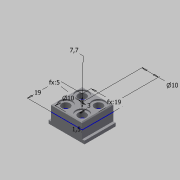
# Autodesk Inventor part: Bumper_button
Saved by Autodesk Inventor 2019.3 (Build 233278000, 278)
## iProperties
Created: 2019-02-26
Part Number: Bumper_button
Material: Generic
Document SubType Name: Modeling
Designer: Varga Daniel
Density: 1 g/cm^3
Appearance: Default
Author: Varga Daniel
Autodesk Inventor part; units mm, degrees
ref_plane "YZ Plane" through (0, 0, 0) normal (1, 0, 0) x (0, 1, 0)
ref_plane "XZ Plane" through (0, 0, 0) normal (0, 1, 0) x (-1, 0, 0)
ref_plane "XY Plane" through (0, 0, 0) normal (0, 0, 1) x (1, 0, 0)
derived "Base_part.ipt"
sketch "Beam_sketch" plane through (0, 0, 0) normal (0, 1, 0) x (-1, 0, 0)
  line L0 (5, 0) -> (25, 0)
  line L1 (30, 5) -> (30, 25)
  line L2 (25, 30) -> (5, 30)
  line L3 (0, 25) -> (0, 5)
  line L4 (5, 29) -> (25, 29)
  line L5 (29, 25) -> (29, 5)
  line L6 (25, 1) -> (5, 1)
  line L7 (1, 5) -> (1, 25)
  circle A0 centre (5, 5) radius 2.5
  circle A1 centre (5, 5) radius 3.5
  arc A2 (25, 0) -> (30, 5) centre (25, 5) ccw
  arc A3 (30, 25) -> (25, 30) centre (25, 25) ccw
  arc A4 (5, 30) -> (0, 25) centre (5, 25) ccw
  arc A5 (0, 5) -> (5, 0) centre (5, 5) ccw
  arc A6 (1, 5) -> (5, 1) centre (5, 5) ccw
  arc A7 (5, 29) -> (1, 25) centre (5, 25) ccw
  arc A8 (29, 25) -> (25, 29) centre (25, 25) ccw
  arc A9 (25, 1) -> (29, 5) centre (25, 5) ccw
  line L8 (49.1041, 15) -> (-27.081, 15) construction
  line L9 (31.1478, 10) -> (-2.4877, 10) construction
  line L10 (-2.8604, 5) -> (35.495, 5) construction
  line L11 (5, -2.5736) -> (5, 36.7522) construction
  line L12 (15, -1.4978) -> (15, 34.8784) construction
  line L13 (1.5359, 5.5) -> (1, 5.5)
  line L14 (1.5359, 4.5) -> (1.0314, 4.5)
  line L15 (28.9686, 4.5) -> (8.4641, 4.5)
  line L16 (29, 5.5) -> (8.4641, 5.5)
  line L17 (4.5, 1.5359) -> (4.5, 1.0314)
  line L18 (5.5, 1.5359) -> (5.5, 1)
  line L19 (29, 10.5) -> (1, 10.5)
  line L20 (29, 9.5) -> (1, 9.5)
  line L21 (4.5, 28.9686) -> (4.5, 10.5)
  line L22 (4.5, 9.5) -> (4.5, 8.4641)
  line L23 (5.5, 29) -> (5.5, 10.5)
  line L24 (5.5, 9.5) -> (5.5, 8.4641)
  point P0 (0, 0)
  point P1 (30, 30)
  point P2 (0, 30)
  dimension "d4" = 7
  dimension "d3" = 5
  dimension "d5" = 1
  measures "d3" diameter of A0
  measures "d5" distance between parallel lines of L3 L7
sketch "Sketch1" plane through (0, 0, 0) normal (0, 1, 0) x (-1, 0, 0)
  line L0 (9.5, -9.5) -> (-9.5, -9.5)
  line L1 (-9.5, -9.5) -> (-9.5, 9.5)
  line L2 (-9.5, 9.5) -> (9.5, 9.5)
  line L3 (9.5, 9.5) -> (9.5, -9.5)
  line L4 (9.5, -9.5) -> (-9.5, 9.5) construction
  line L5 (-9.5, -9.5) -> (9.5, 9.5) construction
  line L6 (0, -9.5) -> (0, 9.5) construction
  line L7 (9.5, 0) -> (-9.5, 0) construction
  circle A0 centre (5, -5) radius 3.85
  circle A1 centre (5, -5) radius 2.5
  circle A2 centre (-5, -5) radius 3.85
  circle A3 centre (-5, -5) radius 2.5
  circle A4 centre (5, 5) radius 3.85
  circle A5 centre (5, 5) radius 2.5
  circle A6 centre (-5, 5) radius 3.85
  circle A7 centre (-5, 5) radius 2.5
  line L8 (-8, 8) -> (-8, -8)
  line L9 (-8, -8) -> (8, -8)
  line L10 (8, -8) -> (8, 8)
  line L11 (8, 8) -> (-8, 8)
  circle A8 centre (0, 0) radius 1.5
  dimension "d0" = 19
  dimension "d1" = 19
  dimension "d6" = 10
  dimension "d7" = 5
  dimension "d8" = 7.7
  dimension "d9" = 10
  dimension "d22" = 1.5
  dimension "d25" = 3
  constraints: 24 end point, 9 centre point, 6 midpoint, 6 symmetric about line, 5 coincident, 4 parallel, 2 perpendicular, 1 horizontal, 9 other
  measures "d0" distance between parallel lines of L2 L0
  measures "d1" distance between parallel lines of L1 L3
  measures "d6" diameter of A0.centre L7
  measures "d7" diameter of A1
  measures "d8" diameter of A0
  measures "d9" diameter of A1.centre L6
  measures "d22" distance between parallel lines of L8 L1
  measures "d25" diameter of A8
extrude "Extrusion1" add sketch "Sketch1" along normal blind 4 contours L0 L1 L2 L3 | A0 L10 | L10 A0 L9 | A0 L9 A2 L8 A6 L11 A4 L10 | L10 L9 A0 | L9 A0 | L10 A4 | A4 L11 L10 | L9 A2 L8 | A2 L9 | A4 L11 | A4 L11 L10 | L9 L8 A2 | L11 A6 | A6 L8 L11 | A2 L8 | A6 L8 L11 | A6 L8 | A8
extrude "Extrusion2" cut sketch "Sketch1" against normal blind 0.8 from surface at 4 contours A0 L10 | L10 A0 L9 | L9 A0 | L10 A4 | A4 L11 L10 | L9 A2 L8 | A2 L9 | A4 L11 | L11 A6 | A6 L8 L11 | A2 L8 | A6 L8 picked at (5.1004, -7.8273) picked at (4.8996, 7.8273) picked at (-5.1004, -7.8273) picked at (-5.1004, 7.8273)
chamfer "Chamfer2" distance 0.5 angle 45 4 edges at (-9.5, 4, 0) (0, 4, -9.5) (9.5, 4, 0) (0, 4, 9.5)
extrude "Extrusion3" add sketch "Sketch1" against normal blind 8.4 from surface at 3.2 contours A0 L10 | L10 A0 L9 | L9 A0 | L10 A4 | A4 L11 L10 | L9 A2 L8 | A2 L9 | A4 L11 | L11 A6 | A6 L8 L11 | A2 L8 | A6 L8 picked at (5.1004, -7.8273) picked at (4.8996, 7.8273) picked at (-5.1004, -7.8273) picked at (-5.1004, 7.8273)
extrude "Extrusion4" add sketch "Sketch1" against normal blind 7 contours L0 L1 L2 L3
extrude "Extrusion5" add sketch "Sketch1" against normal blind 5 contours A8
sketch "Sketch3" plane through (9.5, 3.5, -9.5) normal (0, 0, -1) x (-1, 0, 0)
  line L0 (0, 0) -> (0, -10.5) projected
  line L1 (19, -10.5) -> (19, 0) projected
  line L2 (0, -10.5) -> (-1.45, -10.5)
  line L3 (-1.45, -10.5) -> (-1.45, -8.5443)
  line L4 (-1.45, -8.5443) -> (0, -8.5443)
  line L5 (0, -8.5443) -> (0, -10.5)
  line L6 (19, -10.5) -> (20.45, -10.5)
  line L7 (20.45, -10.5) -> (20.45, -8.5443)
  line L8 (20.45, -8.5443) -> (19, -8.5443)
  line L9 (19, -8.5443) -> (19, -10.5)
  line L10 (19, -10.5) -> (0, -10.5) projected
  line L11 (0, 0) -> (19, 0) projected
  point P0 (9.5, -3.5)
  dimension "d28" = 1.45
  dimension "d30" = 1.45
  constraints: 16 end point, 4 parallel, 3 collinear, 2 horizontal, 2 perpendicular
  measures "d28" distance between parallel lines of L3 L0
  measures "d30" distance between parallel lines of L7 L1
extrude "Extrusion6" add sketch "Sketch3" against normal up to surface (19 mm away) contours L0 L2 L3 L4 | L8 L7 L6 L1
equation "\"d1\" = d0"
equation "\"d7\" = d3"
equation "\"d20\" = Hole_height"
equation "\"d30\" = d28"
equation "\"Hole_height\" = 8.4"
body "Solid1"
